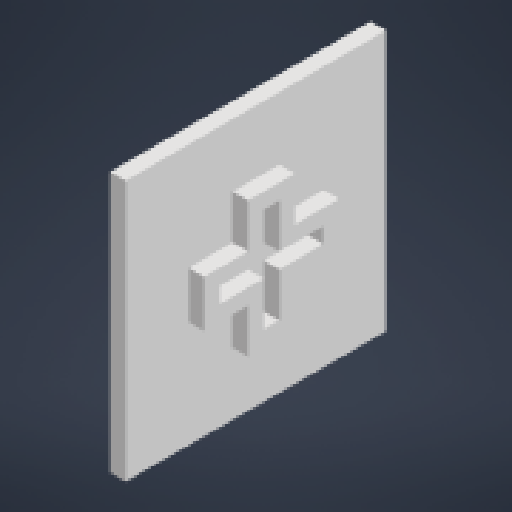
# Autodesk Inventor part: Reflector
Saved by Autodesk Inventor 2027 (Build 310192000, 192)
## iProperties
Created: 2026-03-30
Part Number: Reflector
Material: Generic
Document SubType Name: Modeling
Designer: Tueha
Density: 1 g/cm^3
Appearance: Default
Author: Tueha
Autodesk Inventor part; units mm, degrees
ref_plane "YZ Plane" through (0, 0, 0) normal (1, 0, 0) x (0, 1, 0)
ref_plane "XZ Plane" through (0, 0, 0) normal (0, 1, 0) x (-1, 0, 0)
ref_plane "XY Plane" through (0, 0, 0) normal (0, 0, 1) x (1, 0, 0)
sketch "Sketch3" plane through (0, 0, 0) normal (1, 0, 0) x (0, 1, 0)
  line L0 (0, 0) -> (-75, 0)
  line L1 (-75, 0) -> (-75, -75)
  line L2 (-75, -75) -> (0, -75)
  line L3 (0, -75) -> (0, 0)
  dimension "d0" = 75
  dimension "d1" = 75
  constraints: 8 end point, 2 parallel, 1 horizontal, 1 perpendicular
  measures "d0" distance of L1.end L2.end
  measures "d1" distance of L0.end L1.end
extrude "Extrusion1" add sketch "Sketch3" along normal blind 6
sketch "Sketch5" plane through (6, 0, 0) normal (1, 0, 0) x (0, 0, -1)
  circle A0 centre (12.7921, -17.6697) radius 1.5
  point P0 (0, 0)
  dimension "d27" = 3
  constraints: 1 centre point
  measures "d27" diameter of A0
extrude "Extrusion3" cut sketch "Sketch5" against normal blind 8.2875
equation "\"d0\" = d1"
body "Solid1"
